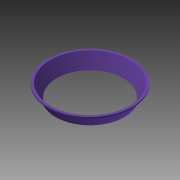
# Autodesk Inventor part: base plate cone
Saved by Autodesk Inventor 2015 (Build 190159000, 159)
## iProperties
Created: 2015-10-21
Part Number: base plate cone
Material: Polyethylene, High Density
Document SubType Name: Modeling
Designer: dagmawi
Density: 0.952 g/cm^3
Appearance: Violet
Author: dagmawi
Autodesk Inventor part; units mm, degrees
ref_plane "YZ Plane" through (0, 0, 0) normal (1, 0, 0) x (0, 1, 0)
ref_plane "XZ Plane" through (0, 0, 0) normal (0, 1, 0) x (-1, 0, 0)
ref_plane "XY Plane" through (0, 0, 0) normal (0, 0, 1) x (1, 0, 0)
sketch "Sketch1" plane through (0, 0, 0) normal (1, 0, 0) x (0, 1, 0)
  line L0 (4.3395, -43.3832) -> (20.7479, -51.7652)
  line L1 (-4.1496, 0) -> (24.8975, 0) projected
  line L2 (20.7479, -51.7652) -> (20.7479, -54.9402)
  line L3 (4.3395, -43.3832) -> (4.3395, -44.9707)
  line L4 (4.3395, -44.9707) -> (19.1604, -52.5417)
  line L5 (20.7479, -54.9402) -> (19.1604, -54.9402)
  line L6 (19.1604, -54.9402) -> (19.1604, -52.5417)
  point P0 (0, 0)
  dimension "d1" = 51.7652
  dimension "d3" = 3.175
  dimension "d5" = 1.5875
  constraints: 12 end point, 2 vertical, 1 horizontal, 1 parallel
  measures "d1" distance from line of L0.end L1
  measures "d3" distance of L0.end L2.end
  measures "d5" distance of L2.end L5.end
revolve "Revolution1" add sketch "Sketch1" angle 360 about axis through (0, -10, 0) along (0, 1, 0)
body "Solid1"
